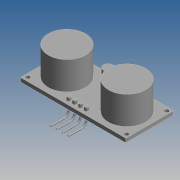
# Autodesk Inventor part: FE014
Saved by Autodesk Inventor 2015 SP1 (Build 190203100, 203)
## iProperties
Created: 2014-10-07
Part Number: FE014
Material: Fourniture / Geliefertes
Document SubType Name: Modeling
Designer: grp
Density: 1 g/cm^3
Appearance: Par défaut
Description: Capteur ultrason
Author: grp
Autodesk Inventor part; units mm, degrees
ref_plane "YZ Plane" through (0, 0, 0) normal (1, 0, 0) x (0, 1, 0)
ref_plane "XZ Plane" through (0, 0, 0) normal (0, 1, 0) x (-1, 0, 0)
ref_plane "XY Plane" through (0, 0, 0) normal (0, 0, 1) x (1, 0, 0)
sketch "Sketch1" plane through (0, 0, 0) normal (0, 0, 1) x (1, 0, 0)
  line L0 (0, 0) -> (45.2, 0)
  line L1 (45.2, 0) -> (45.2, 20.5)
  line L2 (45.2, 20.5) -> (0, 20.5)
  line L3 (0, 20.5) -> (0, 0)
  dimension "d0" = 45.2
  dimension "d1" = 20.5
  constraints: 8 end point, 2 parallel, 1 horizontal, 1 perpendicular
  measures "d0" distance of L2.end L1.end
  measures "d1" distance of L1.end L0.end
extrude "Extrusion1" add sketch "Sketch1" along normal blind 6
sketch "Esquisse2" plane through (0, 0, 6) normal (0, 0, 1) x (1, 0, 0)
  line L0 (0, 0) -> (45.2, 0) construction
  line L1 (45.2, 0) -> (45.2, 20.5) construction
  line L2 (45.2, 20.5) -> (0, 20.5) construction
  line L3 (0, 20.5) -> (0, 0) construction
  line L4 (22.6, 20.5) -> (22.6, 0) construction
  line L5 (18.85, 2) -> (26.35, 2) construction
  circle A0 centre (26.35, 2) radius 0.75
  circle A1 centre (23.85, 2) radius 0.75
  circle A2 centre (21.35, 2) radius 0.75
  circle A3 centre (18.85, 2) radius 0.75
  dimension "d4" = 7.5
  dimension "d5" = 3.75
  dimension "d6" = 2
  dimension "d7" = 1.5
  dimension "d10" = 2.5
  constraints: 4 centre point, 4 end point, 2 horizontal, 2 midpoint, 1 coincident, 6 other
  measures "d4" distance of L5.start L5.end
  measures "d5" distance from line of L4 L5.start
  measures "d6" distance between parallel lines of L5 L0
  measures "d7" diameter of A0
  measures "d10" distance of A0.centre A1.centre
extrude "Extrusion2" add sketch "Esquisse2" along normal blind 1.5
sketch "Esquisse3" plane through (0, 0, 0) normal (0, -1, 0) x (1, 0, 0)
  line L0 (0, 0) -> (45.2, 0) construction
  line L1 (45.2, 0) -> (45.2, 6) construction
  line L2 (0, 6) -> (45.2, 6) construction
  line L3 (0, 0) -> (0, 6) construction
  line L4 (27.1, 7.5) -> (25.6, 7.5) construction
  line L5 (24.6, 7.5) -> (23.1, 7.5) construction
  line L6 (22.1, 7.5) -> (20.6, 7.5) construction
  line L7 (19.6, 7.5) -> (18.1, 7.5) construction
  line L8 (26.35, 7.5) -> (26.35, 0) construction
  line L9 (23.85, 7.5) -> (23.85, 0) construction
  line L10 (21.35, 7.5) -> (21.35, 0) construction
  line L11 (18.85, 7.5) -> (18.85, 0) construction
  line L12 (14.526, 0.4) -> (30.2694, 0.4) construction
  circle A0 centre (26.35, 0.4) radius 0.4
  circle A1 centre (23.85, 0.4) radius 0.4
  circle A2 centre (21.35, 0.4) radius 0.4
  circle A3 centre (18.85, 0.4) radius 0.4
  dimension "d17" = 0.4
  constraints: 12 point on line, 10 end point, 4 midpoint, 4 perpendicular, 4 vertical alignment, 1 horizontal, 8 other
  measures "d17" distance between parallel lines of L0 L12
extrude "Extrusion3" add sketch "Esquisse3" along normal blind 6
fillet "Congé1" radius 0.3 4 edges at (18.45, -6, 0.4) (20.95, -6, 0.4) (23.45, -6, 0.4) (25.95, -6, 0.4)
sketch "Esquisse4" plane through (0, 0, 6) normal (0, 0, 1) x (1, 0, 0)
  circle A0 centre (21.35, 2) radius 0.75 construction
  circle A1 centre (26.35, 2) radius 0.75 construction
  circle A2 centre (23.85, 2) radius 0.75 construction
  circle A3 centre (18.85, 2) radius 0.75 construction
  line L0 (0, 0) -> (45.2, 0) construction
  line L1 (45.2, 0) -> (45.2, 20.5) construction
  line L2 (45.2, 20.5) -> (0, 20.5) construction
  line L3 (0, 20.5) -> (0, 0) construction
  line L4 (0, 10.25) -> (45.2, 10.25) construction
  circle A4 centre (9.7, 10.25) radius 8
  circle A5 centre (35.5, 10.25) radius 8
  line L5 (22.6, 20.5) -> (22.6, 0) construction
  dimension "d21" = 16
  dimension "d22" = 16
  dimension "d23" = 25.8
  dimension "d24" = 12.9
  constraints: 4 end point, 4 midpoint, 2 centre point, 2 point on line
  measures "d21" diameter of A4
  measures "d22" diameter of A5
  measures "d23" distance of A5.centre A4.centre
  measures "d24" distance from line of A4.centre L5
extrude "Extrusion4" add sketch "Esquisse4" along normal blind 12
sketch "Esquisse5" plane through (0, 0, 6) normal (0, 0, 1) x (1, 0, 0)
  circle A0 centre (9.7, 10.25) radius 8 construction
  circle A1 centre (35.5, 10.25) radius 8 construction
  circle A2 centre (21.35, 2) radius 0.75 construction
  circle A3 centre (26.35, 2) radius 0.75 construction
  circle A4 centre (23.85, 2) radius 0.75 construction
  circle A5 centre (18.85, 2) radius 0.75 construction
  line L0 (0, 0) -> (45.2, 0) construction
  line L1 (45.2, 0) -> (45.2, 20.5) construction
  line L2 (45.2, 20.5) -> (0, 20.5) construction
  line L3 (0, 20.5) -> (0, 0) construction
  line L4 (22.6, 20.5) -> (22.6, 0) construction
  line L5 (19.1, 18.5) -> (26.1, 18.5) construction
  line L6 (19.1, 18.5) -> (26.1, 18.5) construction
  line L7 (19.1, 16.5) -> (26.1, 16.5)
  line L8 (26.1, 20.5) -> (19.1, 20.5)
  arc A6 (19.1, 20.5) -> (19.1, 16.5) centre (19.1, 18.5) ccw
  arc A7 (26.1, 16.5) -> (26.1, 20.5) centre (26.1, 18.5) ccw
  line L9 (45.2, 20.5) -> (0, 20.5) projected
  point P0 (22.6, 18.5)
  point P1 (22.6, 18.5)
  dimension "d27" = 7
  dimension "d28" = 2
  constraints: 12 end point, 4 midpoint, 4 point on circle, 4 tangent, 2 centre point, 2 equal length, 1 collinear, 1 horizontal, 1 point on line
  measures "d27" distance of L5.start L5.end
  measures "d28" distance between parallel lines of L5 L2
extrude "Extrusion5" add sketch "Esquisse5" along normal blind 4
sketch "Esquisse6" plane through (0, 0, 0) normal (0, 0, -1) x (-1, 0, 0)
  line L0 (0, 0) -> (-18.85, 0) projected
  line L1 (0, 20.5) -> (0, 0) projected
  line L2 (-45.2, 20.5) -> (0, 20.5) projected
  line L3 (-45.2, 0) -> (-45.2, 20.5) projected
  line L4 (-26.35, 0) -> (-45.2, 0) projected
  line L5 (-23.85, 0) -> (-26.35, 0) projected
  line L6 (-21.35, 0) -> (-23.85, 0) projected
  line L7 (-18.85, 0) -> (-21.35, 0) projected
extrude "Extrusion6" cut sketch "Esquisse6" against normal blind 4.3
sketch "Esquisse7" plane through (0, 0, 0) normal (0, 1, 0) x (-1, 0, 0)
  circle A0 centre (-18.85, 0.4) radius 0.4 projected
  circle A1 centre (-23.85, 0.4) radius 0.4 projected
  circle A2 centre (-26.35, 0.4) radius 0.4 projected
  circle A3 centre (-21.35, 0.4) radius 0.4 projected
  line L0 (-16.7562, 2.4) -> (-29.853, 2.4)
  point P0 (0, 0)
  dimension "d33" = 4
  constraints: 2 end point, 1 horizontal
  measures "d33" diameter of A2.centre L0
revolve "Révolution1" add sketch "Esquisse7" angle 90 about axis through (16.7562, 0, 2.4) along (1, 0, 0)
sketch "Esquisse8" plane through (18.85, 2, 2.4) normal (0, 0, 1) x (1, 0, 0)
  circle A0 centre (7.5, 0) radius 0.4 projected
  circle A1 centre (5, 0) radius 0.4 projected
  circle A2 centre (2.5, 0) radius 0.4 projected
  circle A3 centre (0, 0) radius 0.4 projected
  point P0 (-18.85, -2)
extrude "Extrusion7" add sketch "Esquisse8" along normal up to next
sketch "Esquisse9" plane through (0, 0, 4.3) normal (0, 0, -1) x (-1, 0, 0)
  circle A0 centre (-21.35, 2) radius 0.4 construction
  circle A1 centre (-26.35, 2) radius 0.4 construction
  circle A2 centre (-23.85, 2) radius 0.4 construction
  circle A3 centre (-18.85, 2) radius 0.4 construction
  line L0 (0, 0) -> (-45.2, 0) construction
  line L1 (0, 20.5) -> (0, 0) construction
  line L2 (-45.2, 20.5) -> (0, 20.5) construction
  line L3 (-45.2, 0) -> (-45.2, 20.5) construction
  line L4 (0, 10.25) -> (-45.2, 10.25) construction
  line L5 (-22.6, 0) -> (-22.6, 20.5) construction
  line L6 (-1.45, 1.6) -> (-43.75, 1.6) construction
  line L7 (-43.75, 1.6) -> (-43.75, 18.9) construction
  line L8 (-43.75, 18.9) -> (-1.45, 18.9) construction
  line L9 (-1.45, 18.9) -> (-1.45, 1.6) construction
  point P0 (-22.6, 1.6)
  point P1 (-43.75, 10.25)
  dimension "d37" = 17.3
  dimension "d38" = 42.3
  constraints: 12 end point, 6 midpoint, 4 coincident, 2 parallel, 2 point on line, 1 horizontal, 1 perpendicular
  measures "d37" distance of L6.end L7.end
  measures "d38" distance of L7.end L8.end
hole "Perçage1" at (1.45, 1.6, 4.3) at (1.45, 18.9, 4.3) at (43.75, 18.9, 4.3) at (43.75, 1.6, 4.3) direction (0, 0, 1) diameter 1.8 end through all
equation "\"d5\" = 0.5 * d4"
equation "\"d22\" = d21"
equation "\"d24\" = 0.5 * d23"
